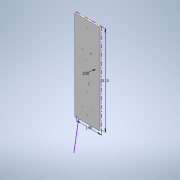
# Autodesk Inventor part: Base Plate
Saved by Autodesk Inventor 2020 (Build 240168000, 168)
## iProperties
Created: 2021-02-01
Part Number: Base Plate
Material: Generic
Document SubType Name: Modeling
Designer: james
Density: 1 g/cm^3
Appearance: Default
Author: james
Autodesk Inventor part; units mm, degrees
ref_plane "YZ Plane" through (0, 0, 0) normal (1, 0, 0) x (0, 1, 0)
ref_plane "XZ Plane" through (0, 0, 0) normal (0, 1, 0) x (-1, 0, 0)
ref_plane "XY Plane" through (0, 0, 0) normal (0, 0, 1) x (1, 0, 0)
sketch "Sketch2" plane through (0, 0, 0) normal (0, 0, 1) x (1, 0, 0)
  line L0 (0.7139, -10.8339) -> (139.63, -10.8339) construction
  line L1 (139.63, -10.8339) -> (139.63, -503.5464) construction
  line L2 (139.63, -503.5464) -> (0.7139, -503.5464) construction
  line L3 (0.7139, -503.5464) -> (0.7139, -10.8339) construction
  line L4 (0, 0) -> (140, 0)
  line L5 (140, 0) -> (140, -515)
  line L6 (140, -515) -> (0, -515)
  line L7 (0, -515) -> (0, 0)
  point P0 (72.592, -40.5851)
  point P1 (90.1811, -155.548)
  point P2 (95.7794, -155.548)
  point P3 (44.0646, -155.548)
  point P4 (62.3487, -199.5395)
  point P5 (78.9817, -308.5348)
  point P6 (78.9817, -314.1345)
  point P7 (73.3117, -356.7556)
  point P8 (100.7597, -430.2294)
  point P9 (73.3117, -471.603)
  point P10 (41.9821, -445.6955)
  dimension "d23" = 140
  dimension "d24" = 515
  constraints: 8 end point, 2 parallel, 1 coincident, 1 horizontal, 1 perpendicular, 2 other
  measures "d23" distance of L5.end L6.end
  measures "d24" distance of L4.end L5.end
extrude "Extrusion1" add sketch "Sketch2" along normal blind 10
hole "Hole1" at (72.592, -40.5851, 0) at (95.7794, -155.548, 0) at (44.0646, -155.548, 0) at (62.3487, -199.5395, 0) at (78.9817, -314.1345, 0) at (73.3117, -356.7556, 0) at (100.7597, -430.2294, 0) at (41.9821, -445.6955, 0) direction (0, 0, 1) diameter 2.5 end through all
hole "Hole2" at (90.1811, -155.548, 0) at (78.9817, -308.5348, 0) at (73.3117, -471.603, 0) direction (0, 0, 1) diameter 4 end through all
sketch "Sketch4" plane through (0, 0, 0) normal (0, 0, -1) x (-1, 0, 0)
  circle A0 centre (-78.9817, -308.5348) radius 2 projected
  circle A1 centre (-90.1811, -155.548) radius 2 projected
  circle A2 centre (-73.3117, -471.603) radius 2 projected
  circle A3 centre (-100.7597, -430.2294) radius 1.25 projected
  circle A4 centre (-78.9817, -314.1345) radius 1.25 projected
  circle A5 centre (-44.0646, -155.548) radius 1.25 projected
  circle A6 centre (-72.592, -40.5851) radius 1.25 projected
  circle A7 centre (-95.7794, -155.548) radius 1.25 projected
  circle A8 centre (-62.3487, -199.5395) radius 1.25 projected
  circle A9 centre (-73.3117, -356.7556) radius 1.25 projected
  circle A10 centre (-41.9821, -445.6955) radius 1.25 projected
  line L0 (-140, -515) -> (-140, 0) projected
  line L1 (0, -515) -> (-140, -515) projected
  line L2 (0, 0) -> (0, -515) projected
  line L3 (-140, 0) -> (0, 0) projected
  circle A11 centre (-90.1811, -155.548) radius 2 projected
  line L4 (-90.1811, -155.548) -> (-51.7202, -155.548) construction
  line L5 (-70.9506, -9.8238) -> (-70, -515)
  line L6 (0, -515) -> (-140, -515) projected
  circle A12 centre (-70.4753, -262.4119) radius 50
  circle A13 centre (-73.3117, -471.603) radius 2 projected
  line L7 (-73.3117, -471.603) -> (-70.3812, -312.4118)
  line L8 (-90.1811, -155.548) -> (-70.5694, -212.412)
  line L9 (-44.0646, -289.2625) -> (17.0359, -707.9815)
  dimension "d65" = 100
  constraints: 10 end point, 3 point on line, 2 midpoint, 2 point on circle, 1 centre point, 1 horizontal
  measures "d65" diameter of A12
equation "\"BendRadius\" = Thickness"
equation "\"BendReliefWidth\" = Thickness"
equation "\"BendReliefDepth\" = 0.5 * Thickness"
equation "\"CornerReliefSize\" = 4 * Thickness"
equation "\"MinimumRemnant\" = 2 * Thickness"
equation "\"TransitionRadius\" = BendRadius"
equation "\"JacobiRadiusSize\" = BendRadius"
equation "\"GapSize\" = Thickness"
equation "\"Thickness\" = 3.175"
body "Solid1"
